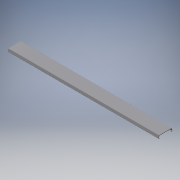
# Autodesk Inventor part: the outside for 2nd slider part
Saved by Autodesk Inventor 2017 (Build 210142000, 142)
## iProperties
Created: 2019-02-04
Part Number: the outside for 2nd slider part
Material: Generic
Document SubType Name: Modeling
Designer: S346852600
Density: 1 g/cm^3
Appearance: Default
Author: S346852600
Autodesk Inventor part; units mm, degrees
ref_plane "YZ Plane" through (0, 0, 0) normal (1, 0, 0) x (0, 1, 0)
ref_plane "XZ Plane" through (0, 0, 0) normal (0, 1, 0) x (-1, 0, 0)
ref_plane "XY Plane" through (0, 0, 0) normal (0, 0, 1) x (1, 0, 0)
sketch "Sketch1" plane through (0, 0, 0) normal (1, 0, 0) x (0, 1, 0)
  line L0 (0, -0.4446) -> (0, -50.3554)
  line L1 (-0.4178, -50.9521) -> (-9.1295, -54.1229)
  line L2 (-9.8331, -53.9343) -> (-12.8126, -50.3834)
  line L3 (-0.4178, 0.1521) -> (-9.1295, 3.3229)
  line L4 (-9.8331, 3.1343) -> (-12.8126, -0.4166)
  line L5 (-11.256, -49.0773) -> (-9.1911, -51.5382)
  line L6 (-8.4874, -51.7268) -> (-2.4498, -49.5293)
  line L7 (-2.032, -48.9325) -> (-2.032, -1.8675)
  line L8 (-2.4498, -1.2707) -> (-8.4874, 0.9268)
  line L9 (-9.1911, 0.7382) -> (-11.256, -1.7227)
  line L10 (-12.8126, -0.4166) -> (-11.256, -1.7227)
  line L11 (-11.256, -49.0773) -> (-12.8126, -50.3834)
  arc A0 (0, -0.4446) -> (-0.4178, 0.1521) centre (-0.635, -0.4446) ccw
  arc A1 (-2.032, -1.8675) -> (-2.4498, -1.2707) centre (-2.667, -1.8675) ccw
  arc A2 (-9.1295, 3.3229) -> (-9.8331, 3.1343) centre (-9.3466, 2.7261) ccw
  arc A3 (-8.4874, 0.9268) -> (-9.1911, 0.7382) centre (-8.7046, 0.3301) ccw
  arc A4 (-2.4498, -49.5293) -> (-2.032, -48.9325) centre (-2.667, -48.9325) ccw
  arc A5 (-0.4178, -50.9521) -> (0, -50.3554) centre (-0.635, -50.3554) ccw
  arc A6 (-9.1911, -51.5382) -> (-8.4874, -51.7268) centre (-8.7046, -51.1301) ccw
  arc A7 (-9.8331, -53.9343) -> (-9.1295, -54.1229) centre (-9.3466, -53.5261) ccw
  point P0 (0, 0)
  point P1 (0, -50.8)
  point P2 (-9.5473, -54.2749)
  point P3 (-9.5473, 3.4749)
  dimension "d0" = 50.8
  dimension "d1" = 10.16
  dimension "d2" = 5.08
  dimension "d3" = 110
  dimension "d4" = 110
  dimension "d5" = 10.16
  dimension "d6" = 5.08
  dimension "d7" = 110
  dimension "d8" = 110
  dimension "d9" = 2.032
  dimension "d10" = 0.635
  constraints: 24 end point, 16 point on circle, 16 tangent, 8 centre point, 8 point on line, 7 equal radius, 1 perpendicular, 1 vertical, 4 other
  measures "d0" distance of point (0, 0) point (0, -50.8)
  measures "d1" distance of point (0, -50.8) point (-9.547, -54.275)
  measures "d2" distance of point (-9.547, -54.275) L2.end
  measures "d3" angle of L0 L1
  measures "d4" angle of L2 L1
  measures "d5" distance of point (0, 0) point (-9.547, 3.475)
  measures "d6" distance of point (-9.547, 3.475) L4.end
  measures "d7" angle of L0 L3
  measures "d8" angle of L4 L3
  measures "d9" distance between parallel lines of L0 L7
  measures "d10" radius of A0
extrude "Extrusion1" add sketch "Sketch1" along normal blind 609.6
body "Solid1"
